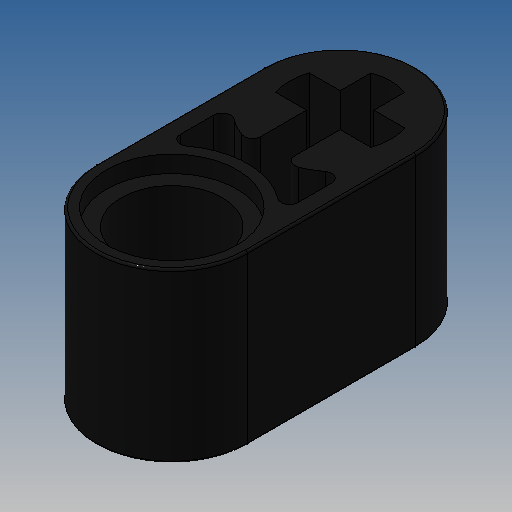
# Autodesk Inventor part: 60483-Black
Saved by Autodesk Inventor 2025 (Build 290162010, 162A)
## iProperties
Created: 2012-03-21
Part Number: 60483-Black
Document SubType Name: Modeling
Designer: D. Kohfeld
Density: 1.06 g/cm^3
Material: ABS Plastic
Mass: 0.464978 g
Surface Area: 8.10321 cm^2
Volume: 0.438658 cm^3
Appearance: Black
Author: D. Kohfeld
Autodesk Inventor part; units mm, degrees
ref_plane "YZ Plane" through (0, 0, 0) normal (1, 0, 0) x (0, 1, 0)
ref_plane "XZ Plane" through (0, 0, 0) normal (0, 1, 0) x (-1, 0, 0)
ref_plane "XY Plane" through (0, 0, 0) normal (0, 0, 1) x (1, 0, 0)
sketch "Sketch1" plane through (0, 0, 0) normal (0, 0, 1) x (1, 0, 0)
  line L0 (3.6, 0) -> (3.6, 8)
  line L1 (-3.6, 8) -> (-3.6, 0)
  arc A0 (3.6, 8) -> (-3.6, 8) centre (0, 8) ccw
  circle A1 centre (0, 8) radius 2.4 construction
  circle A2 centre (0, 8) radius 3.2 construction
  circle A3 centre (0, 0) radius 3.2
  circle A4 centre (0, 0) radius 2.4
  line L2 (0, 0) -> (0, 8) construction
  line L3 (-2.8, 5.7373) -> (-2.8, 2.2627)
  line L4 (2.8, 5.7373) -> (2.8, 2.2627)
  arc A5 (-2.8, 5.7373) -> (2.8, 5.7373) centre (0, 8) ccw
  arc A6 (2.8, 2.2627) -> (-2.8, 2.2627) centre (0, 0) ccw
  arc A7 (-3.6, 0) -> (3.6, 0) centre (0, 0) ccw
  line L5 (0.8, 4.49) -> (0.8, 7.2)
  line L6 (0.8, 7.2) -> (2.2627, 7.2)
  line L7 (2.2627, 8.8) -> (0.8, 8.8)
  line L8 (0.8, 8.8) -> (0.8, 10.2627)
  line L9 (-0.8, 10.2627) -> (-0.8, 8.8)
  line L10 (-0.8, 8.8) -> (-2.2627, 8.8)
  line L11 (-2.2627, 7.2) -> (-0.8, 7.2)
  line L12 (-0.8, 7.2) -> (-0.8, 4.49)
  arc A8 (-2.2627, 8.8) -> (-2.2627, 7.2) centre (0, 8) ccw
  arc A9 (0.8, 10.2627) -> (-0.8, 10.2627) centre (0, 8) ccw
  arc A10 (2.2627, 7.2) -> (2.2627, 8.8) centre (0, 8) ccw
  dimension "d8" = 4.8
  dimension "d9" = 6.4
  dimension "d32" = 7.2
  dimension "d34" = 8
  dimension "d36" = 0.8
  dimension "d52" = 1.6
  constraints: 26 end point, 22 point on circle, 11 centre point, 7 coincident, 7 equal length, 7 equal radius, 5 parallel, 4 tangent, 4 vertical, 3 perpendicular, 1 vertical alignment
  measures "d8" diameter of A1
  measures "d9" diameter of A2
  measures "d32" diameter of A0
  measures "d34" distance of L2.start L2.end
  measures "d36" distance between parallel lines of L1 L3
  measures "d52" distance between parallel lines of L8 L9
extrude "Extrusion1" add sketch "Sketch1" along normal mid plane 8 contours A7 L1 A0 L0 | A3
sketch "Sketch6" plane through (0, 0, 4) normal (0, 0, 1) x (1, 0, 0)
  circle A0 centre (0, 0) radius 3.1
  circle A1 centre (0, 0) radius 2.4 projected
  dimension "d53" = 6.2
  constraints: 1 centre point, 1 concentric
  measures "d53" diameter of A0
extrude "Extrusion7" cut sketch "Sketch6" against normal blind 0.8 contours A0 | A1
mirror "Mirror1" about plane through (0, 0, 0) normal (0, 0, 1) of "Extrusion7"
fillet "Fillet1" radius 0.1 6 edges at (0, 11.6, 4) (3.6, 4, 4) (-3.6, 4, 4) (0, 11.6, -4) (-3.6, 4, -4) (3.6, 4, -4)
fillet "Fillet1" radius 0.4 6 edges at (-2.8, 5.7373, 0) (-2.8, 2.2627, 0) (2.8, 2.2627, 0) (2.8, 5.7373, 0) (0.8, 4.49, 0) (-0.8, 4.49, 0)
equation "\"d8\" = kd"
equation "\"d9\" = tsd"
equation "\"d32\" = tlad"
equation "\"d34\" = lu"
equation "\"d52\" = axlet"
equation "\"d14\" = lu"
equation "\"d41\" = tsl"
equation "\"d45\" = lf"
equation "\"d46\" = tf"
equation "\"kd\" = 4.8"
equation "\"tsd\" = 6.4"
equation "\"tlad\" = 7.2"
equation "\"lu\" = 8"
equation "\"axlet\" = 1.6"
equation "\"tsl\" = 0.8"
equation "\"lf\" = 0.1"
equation "\"tf\" = 0.4"
body "Solid1"
